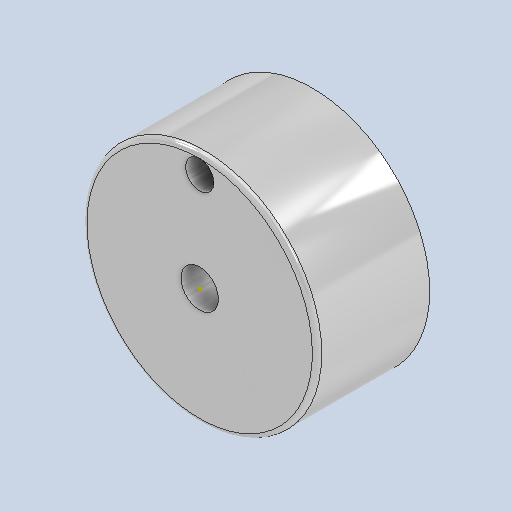
# Autodesk Inventor part: crank_wheel
Saved by Autodesk Inventor 2022.2 (Build 262287010, 287A)
## iProperties
Created: 2022-05-04
Part Number: crank_wheel
Material: Aluminum 6061-AHC
Document SubType Name: Modeling
Designer: 19710060
Density: 2.7 g/cm^3
Appearance: Aluminum - Dark
Author: 19710060
Autodesk Inventor part; units mm, degrees
ref_plane "YZ Plane" through (0, 0, 0) normal (1, 0, 0) x (0, 1, 0)
ref_plane "XZ Plane" through (0, 0, 0) normal (0, 1, 0) x (-1, 0, 0)
ref_plane "XY Plane" through (0, 0, 0) normal (0, 0, 1) x (1, 0, 0)
sketch "Esboço1" plane through (0, 0, 0) normal (0, 0, 1) x (1, 0, 0)
  circle A0 centre (0, 0) radius 12.5
  circle A1 centre (0, 0) radius 2
  dimension "d0" = 25
  dimension "d1" = 4
  constraints: 2 centre point, 2 coincident
  measures "d0" diameter of A0
  measures "d1" diameter of A1
extrude "Extrusão1" add sketch "Esboço1" against normal blind 12
sketch "Esboço2" plane through (0, 0, 0) normal (0, 0, 1) x (1, 0, 0)
  point P0 (0, 0)
fillet "Arredondamento1" radius 0.5 1 edges at (-12.5, 0, 0)
sketch "Esboço3" plane through (0, 0, 0) normal (0, 0, 1) x (1, 0, 0)
  circle A0 centre (0, 10.5) radius 1.5
  circle A1 centre (0, 0) radius 12 projected
  dimension "d5" = 3
  constraints: 1 centre point, 1 tangent
  measures "d5" diameter of A0
extrude "Extrusão2" cut sketch "Esboço3" against normal blind 12 contours A0
